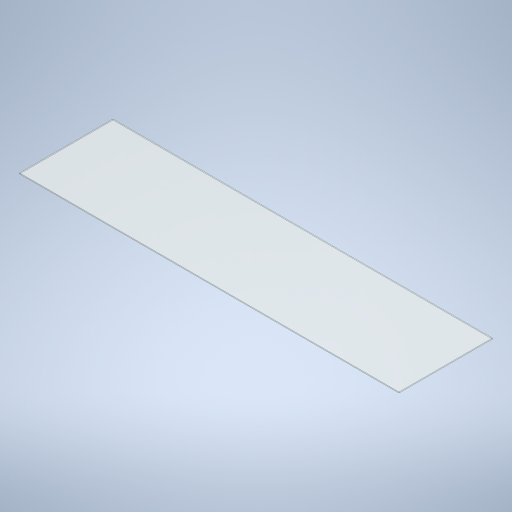
# Autodesk Inventor part: Second_Ceiling
Saved by Autodesk Inventor 2024 (Build 280153000, 153)
## iProperties
Created: 2023-05-20
Part Number: Second_Ceiling
Material: Concrete
Document SubType Name: Modeling
Designer: Tom
Density: 2.40731 g/cm^3
Appearance: Clear
Author: Tom
Autodesk Inventor part; units mm, degrees
ref_plane "YZ Plane" through (0, 0, 0) normal (1, 0, 0) x (0, 1, 0)
ref_plane "XZ Plane" through (0, 0, 0) normal (0, 1, 0) x (-1, 0, 0)
ref_plane "XY Plane" through (0, 0, 0) normal (0, 0, 1) x (1, 0, 0)
sketch "Sketch1" plane through (0, 0, 0) normal (0, 1, 0) x (-1, 0, 0)
  line L0 (-3702.05, 911.6949) -> (3702.05, 911.6949)
  line L1 (3702.05, 911.6949) -> (3702.05, -911.6949)
  line L2 (3702.05, -911.6949) -> (-3702.05, -911.6949)
  line L3 (-3702.05, -911.6949) -> (-3702.05, 911.6949)
  line L4 (0, -911.6949) -> (0, 911.6949)
  line L5 (-3702.05, 0) -> (3702.05, 0)
  point P0 (0, 0)
  point P1 (0, 0)
  dimension "d2" = 1823.3898
  dimension "d3" = 7404.1
  constraints: 12 end point, 5 midpoint, 2 parallel, 1 coincident, 1 horizontal, 1 perpendicular
  measures "d2" distance of L2.end L0.start
  measures "d3" distance of L0.start L0.end
extrude "Extrusion1" add sketch "Sketch1" along normal blind 19.05
body "Solid1"
